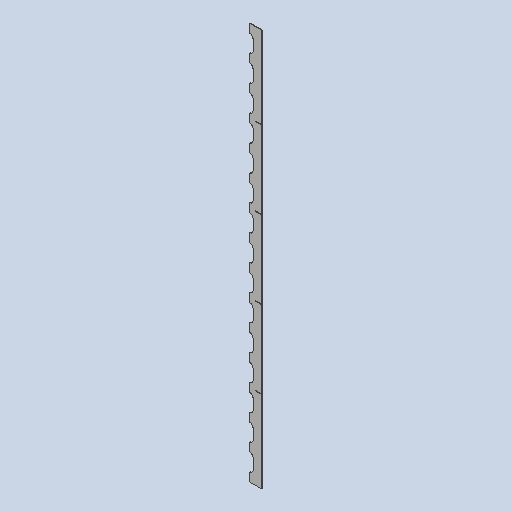
# Autodesk Inventor part: BSH 039 stringer butt end in
Saved by Autodesk Inventor 2025 (Build 290162010, 162A)
## iProperties
Created: 2024-07-23
Part Number: BSH 039 stringer butt end in
Material: 09g2s
Document SubType Name: Sheet Metal
Designer: admin
Density: 7.85 g/cm^3
Sheet Metal Rule: AISI304 3mm Die 32
Sheet Metal Width: 70,289 mm
Sheet Metal Length: 2300,000 mm
Sheet Metal Area: 161664,906 mm^2
Appearance: Default
Mass: 3171.2 g
Surface Area: 2845.67 cm^2
Volume: 403.975 cm^3
Flat Pattern Width: 7.02891 cm
Flat Pattern Length: 230 cm
Flat Pattern Area: 1616.65 cm^2
Stock Number: БШК 039 стрингер торец внутренний
Author: admin
Autodesk Inventor part; units mm, degrees
ref_plane "YZ Plane" through (0, 0, 0) normal (1, 0, 0) x (0, 1, 0)
ref_plane "XZ Plane" through (0, 0, 0) normal (0, 1, 0) x (-1, 0, 0)
ref_plane "XY Plane" through (0, 0, 0) normal (0, 0, 1) x (1, 0, 0)
sketch "Sketch6" plane through (0, 0, 0) normal (0, 1, 0) x (-1, 0, 0)
  line L0 (0, -1150) -> (-70.2891, -1150)
  line L1 (-70.2891, -1150) -> (-70.2891, 1150)
  line L2 (-70.2891, 1150) -> (0, 1150)
  line L3 (0, 1150) -> (0, -1150)
  point P0 (0, 0)
  point P1 (0, 0)
  dimension "d26" = 70.2891
  dimension "d27" = 2300
  measures "d26" distance of L1.end L2.end
  measures "d27" distance of L0.end L1.end
extrude "Plate4" add sketch "Sketch6" along normal blind 3
sketch "Sketch7" plane through (0, 0, 0) normal (0, -1, 0) x (1, 0, 0)
  line L0 (0, 1150) -> (70.2891, 1150) projected
  line L1 (0, -1150) -> (0, 1150) projected
  line L2 (70.2891, -1150) -> (0, -1150) projected
  line L3 (70.2891, 1150) -> (70.2891, -1150) projected
  line L4 (20, -30) -> (20, 30)
  arc A0 (0, -50) -> (20, -30) centre (0, -30) ccw
  arc A1 (20, 30) -> (0, 50) centre (0, 30) ccw
  point P0 (0, 0)
  point P1 (20, 0)
  point P2 (0, 0)
  dimension "d37" = 20
  dimension "d38" = 100
  constraints: 4 point on circle, 4 point on line, 2 centre point, 2 end point, 2 midpoint, 2 tangent, 1 horizontal alignment, 1 vertical
  measures "d37" distance between parallel lines of L1 L4
  measures "d38" distance of A1.end A0.start
extrude "Extrusion2" cut sketch "Sketch7" against normal through all contours A1 L4 A0 L1
pattern_linear "Rectangular Pattern2" count 15 spacing 150 along (0, 0, 1) of "Extrusion2" first direction both ways yes
sketch "Sketch8" plane through (0, 0, 0) normal (0, -1, 0) x (1, 0, 0)
  line L0 (34.2891, 226.6) -> (70.2891, 226.6)
  line L1 (70.2891, 226.6) -> (70.2891, 223.4)
  line L2 (70.2891, 223.4) -> (34.2891, 223.4)
  line L3 (34.2891, 223.4) -> (34.2891, 226.6)
  line L4 (70.2891, 1150) -> (70.2891, -1150) projected
  line L5 (0, 350) -> (0, 400) projected
  line L6 (34.2891, 676.6) -> (70.2891, 676.6)
  line L7 (70.2891, 676.6) -> (70.2891, 673.4)
  line L8 (70.2891, 673.4) -> (34.2891, 673.4)
  line L9 (34.2891, 673.4) -> (34.2891, 676.6)
  line L10 (70.2891, -223.4) -> (34.2891, -223.4)
  line L11 (34.2891, -223.4) -> (34.2891, -226.6)
  line L12 (34.2891, -226.6) -> (70.2891, -226.6)
  line L13 (70.2891, -226.6) -> (70.2891, -223.4)
  line L14 (70.2891, -673.4) -> (34.2891, -673.4)
  line L15 (34.2891, -673.4) -> (34.2891, -676.6)
  line L16 (34.2891, -676.6) -> (70.2891, -676.6)
  line L17 (70.2891, -676.6) -> (70.2891, -673.4)
  point P0 (0, 0)
  point P1 (70.2891, 225)
  point P2 (70.2891, 0)
  point P3 (52.2891, 226.6)
  point P4 (70.2891, 0)
  point P5 (70.2891, 0)
  point P6 (70.2891, 675)
  point P7 (70.2891, 0)
  point P8 (70.2891, -225)
  point P9 (70.2891, 0)
  point P10 (70.2891, -675)
  point P11 (70.2891, 0)
  point P12 (70.2891, 0)
  dimension "d42" = 3.2
  dimension "d44" = 36
  dimension "d45" = 225
  dimension "d46" = 36
  dimension "d47" = 3.2
  dimension "d48" = 450
  dimension "d49" = 36
  dimension "d50" = 36
  dimension "d51" = 3.2
  dimension "d52" = 3.2
  dimension "d53" = 225
  dimension "d54" = 450
  constraints: 32 end point, 8 parallel, 5 midpoint, 4 horizontal, 4 perpendicular, 4 vertical alignment, 8 other
  measures "d42" distance from line of L2 point (52.289, 226.6)
  measures "d44" distance of L1.end L2.end
  measures "d45" distance of point (70.289, 0) point (70.289, 225)
  measures "d46" distance of L7.end L8.end
  measures "d47" distance between parallel lines of L8 L6
  measures "d48" distance of point (70.289, 675) point (70.289, 225)
  measures "d49" distance of L11.end L12.end
  measures "d50" distance of L15.end L16.end
  measures "d51" distance between parallel lines of L14 L16
  measures "d52" distance between parallel lines of L10 L12
  measures "d53" distance of point (70.289, 0) point (70.289, -225)
  measures "d54" distance of point (70.289, -225) point (70.289, -675)
extrude "Extrusion3" cut sketch "Sketch8" against normal through all
equation "\"d53\" = d45"
equation "\"d54\" = d48"
equation "\"d26\" = Stringer3_deep"
equation "\"d46\" = d44"
equation "\"d47\" = d42"
equation "\"d49\" = d44"
equation "\"d50\" = d49"
equation "\"d51\" = d42"
equation "\"d52\" = d42"
equation "\"d28\" = Thickness"
equation "\"BendReliefWidth\" = Thickness"
equation "\"BendReliefDepth\" = 0.5 * Thickness"
equation "\"CornerReliefSize\" = 4 * Thickness"
equation "\"MinimumRemnant\" = 2 * Thickness"
equation "\"TransitionRadius\" = BendRadius"
equation "\"JacobiRadiusSize\" = BendRadius"
equation "\"GapSize\" = Thickness"
equation "\"Stringer3_deep\" = 70.28909"
equation "\"Thickness\" = 3"
equation "\"BendRadius\" = 5"
body "Solid2"
